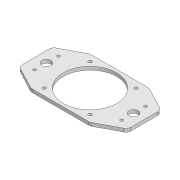
# Autodesk Inventor part: Suporte_inferior_menor
Saved by Autodesk Inventor 2020 (Build 240168000, 168)
## iProperties
Created: 2022-07-20
Part Number: Suporte_inferior_menor
Material: Genérico
Document SubType Name: Modeling
Designer: gabri
Density: 1 g/cm^3
Appearance: Padrão
Author: gabri
Autodesk Inventor part; units mm, degrees
ref_plane "YZ Plane" through (0, 0, 0) normal (1, 0, 0) x (0, 1, 0)
ref_plane "XZ Plane" through (0, 0, 0) normal (0, 1, 0) x (-1, 0, 0)
ref_plane "XY Plane" through (0, 0, 0) normal (0, 0, 1) x (1, 0, 0)
sketch "Esboço1" plane through (0, 0, 0) normal (0, 1, 0) x (-1, 0, 0)
  circle A0 centre (0, 0) radius 32.5
  line L0 (0, 0) -> (36, 0)
  line L1 (36, 0) -> (36, -36)
  line L2 (34.508, -36) -> (0, -36)
  line L3 (0, -36) -> (0, 0)
  circle A1 centre (28, -28) radius 2
  circle A2 centre (53.1, 0) radius 5.5
  circle A3 centre (53.1, -14.5) radius 1.75
  line L4 (66.1814, 0) -> (66.1814, -16.3898)
  line L5 (62.9917, -21.691) -> (37.3183, -35.3012)
  line L6 (66.1814, 0) -> (36, 0)
  arc A4 (62.9917, -21.691) -> (66.1814, -16.3898) centre (60.1814, -16.3898) ccw
  arc A5 (34.508, -36) -> (37.3183, -35.3012) centre (34.508, -30) ccw
  point P0 (32.5, 0)
  point P1 (0, -32.5)
  point P2 (66.1814, -20)
  point P3 (36, -35.8115)
  point P4 (58.6, 0)
  point P5 (47.6, 0)
  dimension "d0" = 65
  dimension "d1" = 36
  dimension "d2" = 36
  dimension "d4" = 4
  dimension "d9" = 11
  dimension "d10" = 17.1
  dimension "d11" = 3.5
  dimension "d12" = 14.5
  dimension "d13" = 20
  dimension "d14" = 6
  dimension "d15" = 6
  dimension "d16" = 30.1814
  constraints: 14 end point, 6 centre point, 4 point on circle, 4 point on line, 4 tangent, 2 horizontal, 2 parallel, 1 coincident, 1 equal radius, 1 perpendicular, 1 vertical
  measures "d0" diameter of A0
  measures "d1" distance of L1.end L2.end
  measures "d2" distance of L1.end L0.end
  measures "d4" diameter of A1
  measures "d9" diameter of A2
  measures "d10" distance from line of A2.centre L1
  measures "d11" diameter of A3
  measures "d12" distance of A3.centre A2.centre
  measures "d13" distance of L4.start point (66.181, -20)
  measures "d14" radius of A4
  measures "d15" radius of A5
  measures "d16" distance between parallel lines of L1 L4
extrude "Extrusão1" add sketch "Esboço1" along normal blind 4 contours L0 L1 A5 L2 L3 A0 | L6 A2 L4 A4 L5 A5 L1
mirror "Espelhamento1" about plane through (0, 0, -32.5) normal (1, 0, 0) of "Extrusão1"
mirror "Espelhamento3" about plane through (47.6, 0, 0) normal (0, 0, 1) of "Extrusão1", "Espelhamento1"
